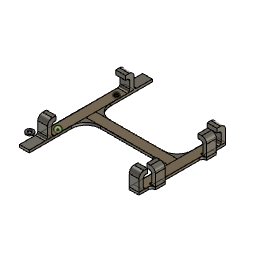
weather_station_battery_holder v17 (Autodesk Fusion 360 design; units mm, degrees)
Autodesk Fusion 360 part; units mm, degrees
sketch "Sketch1" plane through (0, 0, 0) normal (0, 0, 1) x (1, 0, 0)
  circle A0 centre (0, 48) radius 1.5
  circle A1 centre (0, 0) radius 1.5
  line L0 (-5, 59.5) -> (3, 59.5)
  line L1 (3, 59.5) -> (3, -11.5)
  line L2 (3, -11.5) -> (-5, -11.5)
  line L3 (-5, -11.5) -> (-5, 59.5)
  line L4 (-5, 56) -> (3, 56)
  line L5 (-5, -8) -> (3, -8)
  line L6 (3, 20) -> (70, 20)
  line L7 (70, 20) -> (70, 28)
  line L8 (70, 28) -> (3, 28)
  line L9 (3, 28) -> (3, 20)
  line L10 (70, -11.5) -> (78, -11.5)
  line L11 (78, -11.5) -> (78, 59.5)
  line L12 (78, 59.5) -> (70, 59.5)
  line L13 (70, 59.5) -> (70, -11.5)
  line L14 (70, 56) -> (78, 56)
  line L15 (70, -8) -> (78, -8)
  line L16 (78, 49) -> (81, 49)
  line L17 (81, 49) -> (81, 41)
  line L18 (81, 41) -> (78, 41)
  line L19 (78, 41) -> (78, 49)
  line L20 (78, -1) -> (81, -1)
  line L21 (81, -1) -> (81, 7)
  line L22 (81, 7) -> (78, 7)
  line L23 (78, 7) -> (78, -1)
  dimension "d2" = 48
  dimension "d5" = 3
  dimension "d6" = 3
  dimension "d7" = 3
  dimension "d8" = 8
  dimension "d13" = 3.5
  dimension "d14" = 3.5
  dimension "d15" = 8
  dimension "d16" = 20
  dimension "d17" = 8
  dimension "d20" = 83
  dimension "d21" = 3.5
  dimension "d22" = 3.5
  dimension "d23" = 3
  dimension "d24" = 3
  dimension "d25" = 8
  dimension "d26" = 8
  dimension "d36" = 7
  dimension "d37" = 7
  dimension "d86" = 64
  dimension "d87" = 64
  dimension "d89" = 28
  dimension "d90" = 8
  dimension "d91" = 3
  constraint coincident A1.centre origin
  constraint horizontal L0
  constraint vertical L1
  constraint horizontal L2
  constraint vertical L3
  constraint coincident L3 L4.start
  constraint coincident L1 L4.end
  constraint perpendicular L1 L4
  constraint coincident L3 L5.start
  constraint coincident L1 L5.end
  constraint perpendicular L1 L5
  constraint horizontal L6
  constraint vertical L7
  constraint horizontal L8
  constraint vertical L9
  constraint coincident L1 L6.start
  constraint horizontal L10
  constraint vertical L11
  constraint horizontal L12
  constraint vertical L13
  constraint collinear L7 L13
  constraint coincident L13 L14.start
  constraint coincident L11 L14.end
  constraint perpendicular L11 L14
  constraint coincident L13 L15.start
  constraint coincident L11 L15.end
  constraint perpendicular L11 L15
  constraint horizontal L16
  constraint vertical L17
  constraint horizontal L18
  constraint vertical L19
  constraint coincident L11 L16.start
  constraint horizontal L20
  constraint vertical L21
  constraint horizontal L22
  constraint vertical L23
  constraint coincident L11 L20.start
  measures "d2" distance of A1.centre A0.centre
  measures "d5" diameter of A0
  measures "d6" diameter of A1
  measures "d7" distance of A0.centre L1
  measures "d8" distance of L0.start L0.end
  measures "d13" distance of L2 L5
  measures "d14" distance of L0 L4
  measures "d15" distance of L6 L8
  measures "d16" distance of A1.centre L6
  measures "d17" distance of L10.start L10.end
  measures "d20" distance of L2.end L10.end
  measures "d21" distance of L12 L14
  measures "d22" distance of L10 L15
  measures "d23" distance of L21.end L22.end
  measures "d24" distance of L17.end L18.end
  measures "d25" distance of L16.end L17.end
  measures "d26" distance of L20.end L21.end
  measures "d36" distance of L15 L20
  measures "d37" distance of L14 L16
  measures "d86" distance of L14 L15
  measures "d87" distance of L4 L5
  measures "d89" distance of L6 L15
  measures "d90" distance of A0.centre L4
  measures "d91" distance of A1.centre L1
extrude "Extrude1" add sketch "Sketch1" against normal blind 2 contours A0 | A1 | L0 L1 L3 L4 | L1 L3 L4 L5 L9 | L1 L2 L3 L5 | L1 L6 L7 L8 L9 L13 | L7 L11 L13 L14 L15 L19 L23 | L11 L12 L13 L14 | L10 L11 L13 L15 | L11 L16 L17 L18 L19 | L11 L20 L21 L22 L23 makes body 1
extrude "Extrude3" add sketch "Sketch1" along normal blind 10 contours L0 L1 L3 L4 | L1 L2 L3 L5 | L11 L12 L13 L14 | L10 L11 L13 L15 | L11 L16 L17 L18 L19 | L11 L20 L21 L22 L23 bodies 1
sketch "Sketch3" plane through (0, 0, 10) normal (0, 0, 1) x (-1, 0, 0)
  line L0 (5, -59.5) -> (5, -56)
  line L1 (5, -56) -> (-3, -56)
  line L2 (-3, -56) -> (-3, -59.5)
  line L3 (-3, -59.5) -> (5, -59.5)
  line L4 (5, -59.5) -> (-3, -59.5)
  line L5 (-3, -59.5) -> (-3, -52.5)
  line L6 (-3, -52.5) -> (5, -52.5)
  line L7 (5, -52.5) -> (5, -59.5)
  line L8 (-3, 11.5) -> (5, 11.5)
  line L9 (5, 11.5) -> (5, 4.5)
  line L10 (5, 4.5) -> (-3, 4.5)
  line L11 (-3, 4.5) -> (-3, 11.5)
  line L12 (-70, 11.5) -> (-78, 11.5)
  line L13 (-78, 11.5) -> (-78, 4.5)
  line L14 (-78, 4.5) -> (-70, 4.5)
  line L15 (-70, 4.5) -> (-70, 11.5)
  line L16 (-70, -59.5) -> (-78, -59.5)
  line L17 (-78, -59.5) -> (-78, -52.5)
  line L18 (-78, -52.5) -> (-70, -52.5)
  line L19 (-70, -52.5) -> (-70, -59.5)
  line L20 (-81, -49) -> (-73.9864, -49)
  line L21 (-73.9864, -49) -> (-73.9864, -41)
  line L22 (-73.9864, -41) -> (-81, -41)
  line L23 (-81, -41) -> (-81, -49.5224)
  line L24 (-81, -7) -> (-74, -7)
  line L25 (-74, -7) -> (-74, 1)
  line L26 (-74, 1) -> (-81, 1)
  line L27 (-81, 1) -> (-81, -7)
  point P0 (5, 11.5)
  point P1 (-78, -59.5)
  point P2 (-81, -41)
  point P3 (-78, 11.5)
  point P4 (-81, 1)
  point P5 (-70, -59.5)
  point P6 (-70, 11.5)
  point P7 (-81, -49)
  point P8 (-81, -7)
  dimension "d38" = 7
  dimension "d39" = 7
  dimension "d41" = 7
  dimension "d42" = 7
  dimension "d43" = 7
  constraint horizontal L4
  constraint vertical L5
  constraint horizontal L6
  constraint vertical L7
  constraint coincident L0.start L3.end
  constraint horizontal L8
  constraint vertical L9
  constraint horizontal L10
  constraint vertical L11
  constraint horizontal L12
  constraint vertical L13
  constraint horizontal L14
  constraint vertical L15
  constraint horizontal L16
  constraint vertical L17
  constraint horizontal L18
  constraint vertical L19
  constraint horizontal L20
  constraint vertical L21
  constraint horizontal L22
  constraint vertical L23
  constraint horizontal L24
  constraint vertical L25
  constraint horizontal L26
  constraint vertical L27
  constraint coincident P0 L8.end
  constraint coincident P1 L16.end
  constraint coincident P2 L22.end
  constraint coincident P3 L12.end
  constraint coincident P4 L26.end
  constraint coincident P5 L16.start
  constraint coincident P6 L12.start
  constraint coincident P7 L20.start
  constraint coincident P8 L24.start
  measures "d38" distance of P6 L14.end
  measures "d39" distance of P1 L17.end
  measures "d41" distance of P8 L24.end
  measures "d42" distance of L8.start L10.end
  measures "d43" distance of L2.end L5.end
extrude "Extrude4" add sketch "Sketch3" along normal blind 3.5 bodies 1
fillet "Fillet1" radius 12 4 edges at (70, 20, -1) (3, 20, -1) (3, 28, -1) (70, 28, -1) on bodies 1
extrude "Extrude6" cut sketch "Sketch1" against normal blind 7 contours A0 | A1 bodies 1
fillet "Fillet3" radius 2 12 edges at (74, -8, 0) (74, -8, 10) (78, 3, 10) (78, 3, 0) (74, 56, 10) (78, 45, 10) (78, 45, 0) (74, 56, 0) (-1, -8, 10) (-1, -8, 0) (-1, 56, 10) (-1, 56, 0) on bodies 1
thread "Thread6" "ISO Metric profile 3.0 M3x0.5 6H" major diameter 3.086 minor diameter 2.529 pitch 0.5 angle 60 resizes the face on face at (1.4925, -0.1494, -0.6667) on bodies 1
thread "Thread7" "ISO Metric profile 3.0 M3x0.5 6H" major diameter 3.086 minor diameter 2.529 pitch 0.5 angle 60 resizes the face on face at (-1.3822, 47.4173, -1.3333) on bodies 1
sketch "Sketch4" plane through (0, 0, -2) normal (0, 0, -1) x (1, 0, 0)
  circle A0 centre (-11, 0) radius 3
  circle A1 centre (-11, 12) radius 3
  circle A2 centre (-11, 0) radius 1.6
  circle A3 centre (-11, 12) radius 1.6
  circle A4 centre (0, 0) radius 1.2645
  circle A5 centre (0, -48) radius 1.2645
  line L0 (58, -20) -> (15, -20)
  arc A6 (3, -8) -> (15, -20) centre (15, -8) ccw
  line L1 (3, -8) -> (3, 11.5)
  line L2 (3, 11.5) -> (-5, 11.5)
  line L3 (-5, 11.5) -> (-5, -59.5)
  line L4 (-5, -59.5) -> (3, -59.5)
  line L5 (3, -59.5) -> (3, -40)
  arc A7 (15, -28) -> (3, -40) centre (15, -40) ccw
  line L6 (15, -28) -> (58, -28)
  arc A8 (70, -40) -> (58, -28) centre (58, -40) ccw
  line L7 (70, -40) -> (70, -59.5)
  line L8 (70, -59.5) -> (78, -59.5)
  line L9 (78, -59.5) -> (78, -49)
  line L10 (78, -49) -> (81, -49)
  line L11 (81, -49) -> (81, -41)
  line L12 (81, -41) -> (78, -41)
  line L13 (78, -41) -> (78, -7)
  line L14 (78, -7) -> (81, -7)
  line L15 (81, -7) -> (81, 1)
  line L16 (81, 1) -> (78, 1)
  line L17 (78, 1) -> (78, 11.5)
  line L18 (78, 11.5) -> (70, 11.5)
  line L19 (70, 11.5) -> (70, -8)
  arc A9 (58, -20) -> (70, -8) centre (58, -8) ccw
  dimension "d56" = 6
  dimension "d57" = 6
  dimension "d58" = 3.2
  dimension "d59" = 3.2
  constraint concentric A0 A2
  constraint concentric A1 A3
  measures "d56" diameter of A0
  measures "d57" diameter of A1
  measures "d58" diameter of A2
  measures "d59" diameter of A3
extrude "Extrude8" add sketch "Sketch4" against normal blind 1 separate body contours A0 | A1 makes body 2 at (-8.4838, 0.2285, -2) makes body 3 at (-8.4838, -11.7715, -2)
fillet "Fillet4" radius 4 6 edges at (-1, -11.5, 13.5) (-1, 59.5, 13.5) (74, 59.5, 13.5) (81, 45, 13.5) (81, 3, 13.5) (74, -11.5, 13.5) on bodies 1
fillet "Fillet5" radius 3 4 edges at (78, -1, -1) (78, 41, -1) (78, 7, -1) (78, 49, -1) on bodies 1
sketch "Sketch8" plane through (0, 59.5, 0) normal (0, 1, 0) x (-1, 0, 0)
  line L0 (5, 9.5) -> (-3, 9.5)
  line L1 (-3, 9.5) -> (-3, -2)
  line L2 (-3, -2) -> (5, -2)
  line L3 (5, -2) -> (5, 9.5)
  line L4 (-3, -2) -> (5, -2)
  line L5 (5, -2) -> (5, 0)
  line L6 (5, 0) -> (-3, 0)
  line L7 (-3, 0) -> (-3, -2)
  constraint horizontal L4
  constraint vertical L5
  constraint horizontal L6
  constraint vertical L7
  constraint coincident L1.end L2.start
extrude "Extrude12" add sketch "Sketch8" along normal blind 15 contours L1 L2 L3 L4 L5 L6 L7 bodies 1
sketch "Sketch9" plane through (0, -11.5, 0) normal (0, -1, 0) x (1, 0, 0)
  line L0 (3, 9.5) -> (-5, 9.5)
  line L1 (-5, 9.5) -> (-5, -2)
  line L2 (-5, -2) -> (3, -2)
  line L3 (3, -2) -> (3, 9.5)
  line L4 (-5, -2) -> (3, -2)
  line L5 (3, -2) -> (3, 0)
  line L6 (3, 0) -> (-5, 0)
  line L7 (-5, 0) -> (-5, -2)
  constraint horizontal L4
  constraint vertical L5
  constraint horizontal L6
  constraint vertical L7
  constraint coincident L1.end L2.start
extrude "Extrude13" add sketch "Sketch9" along normal blind 15 contours L1 L2 L3 L4 L5 L6 L7 bodies 1
fillet "Fillet9" radius 2 2 edges at (-1, 59.5, 0) (-1, -11.5, 0) on bodies 1
equation "d5 = d6"
equation "d9 = 6.5 mm + d13"
equation "d14 = d13"
equation "d15 = d8"
equation "d16 = ( d2 - d8 ) / 2"
equation "d17 = d8"
equation "d20 = 80 mm + 3 mm"
equation "d21 = d13"
equation "d22 = d13"
equation "d24 = d23"
equation "d26 = d25"
equation "d37 = d36"
equation "d39 = d38"
equation "d42 = d38"
equation "d43 = d38"
equation "d89 = d86 / 2 - d8 / 2"
equation "d90 = ( d87 - d2 ) / 2"
